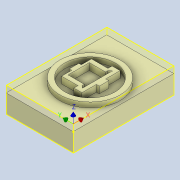
# Autodesk Inventor part: CNC#2 FInal
Saved by Autodesk Inventor 2022 (Build 260153000, 153)
## iProperties
Created: 2022-01-13
Part Number: CNC#2 FInal
Material: Generic
Document SubType Name: Modeling
Designer: student
Density: 1 g/cm^3
Appearance: Default
Author: student
Autodesk Inventor part; units mm, degrees
ref_plane "YZ Plane" through (0, 0, 0) normal (1, 0, 0) x (0, 1, 0)
ref_plane "XZ Plane" through (0, 0, 0) normal (0, 1, 0) x (-1, 0, 0)
ref_plane "XY Plane" through (0, 0, 0) normal (0, 0, 1) x (1, 0, 0)
sketch "Sketch1" plane through (0, 0, 0) normal (0, 1, 0) x (-1, 0, 0)
  line L0 (0, 0) -> (50.8, 0)
  line L1 (50.8, 0) -> (50.8, -76.2)
  line L2 (50.8, -76.2) -> (0, -76.2)
  line L3 (0, -76.2) -> (0, 0)
  dimension "d0" = 50.8
  dimension "d1" = 76.2
  constraints: 8 end point, 2 parallel, 1 horizontal, 1 perpendicular
  measures "d0" distance of L1.end L2.end
  measures "d1" distance of L0.end L1.end
extrude "Extrusion1" add sketch "Sketch1" along normal blind 13.97
sketch "Sketch6" plane through (0, 13.97, 0) normal (0, 1, 0) x (1, 0, 0)
  point P0 (0, 0)
sketch "Sketch7" plane through (0, 13.97, 0) normal (0, 1, 0) x (1, 0, 0)
  point P0 (0, 0)
sketch "Sketch8" plane through (0, 13.97, 0) normal (0, 1, 0) x (1, 0, 0)
  circle A0 centre (-25.4, 38.1) radius 22.86
  circle A1 centre (-25.4, 38.1) radius 19.05
  point P0 (0, 0)
  dimension "d30" = 45.72
  dimension "d31" = 38.1
  constraints: 2 centre point, 1 coincident
  measures "d30" diameter of A0
  measures "d31" diameter of A1
extrude "Extrusion15" add sketch "Sketch8" along normal blind 3.81
sketch "Sketch9" plane through (-25.4, 13.97, -38.1) normal (0, 1, 0) x (1, 0, 0)
  line L0 (-8.6694, 8.1535) -> (3.6792, 8.1535)
  line L1 (3.6792, 8.1535) -> (3.6792, 9.8977)
  line L2 (3.6792, 9.8977) -> (5.4931, 11.4325)
  line L3 (5.4931, 11.4325) -> (5.4931, 0.0971)
  line L4 (-8.6694, 8.1535) -> (-8.6694, 0.0971)
  line L5 (-8.6694, -7.9593) -> (3.6792, -7.9593)
  line L6 (3.6792, -7.9593) -> (3.6792, -9.7035)
  line L7 (3.6792, -9.7035) -> (5.4931, -11.2383)
  line L8 (5.4931, -11.2383) -> (5.4931, 0.0971)
  line L9 (-8.6694, -7.9593) -> (-8.6694, 0.0971)
  line L10 (8.2546, 0.0971) -> (8.2546, -14.3778)
  line L11 (8.2546, -14.3778) -> (2.1623, -14.3778)
  line L12 (2.1623, -14.3778) -> (2.1623, -11.2383)
  line L13 (2.1623, -11.2383) -> (-10.3102, -11.2383)
  line L14 (-10.3102, -11.2383) -> (-10.3102, 0.0971)
  line L15 (8.2546, 0.0971) -> (8.2546, 14.572)
  line L16 (8.2546, 14.572) -> (2.1623, 14.572)
  line L17 (2.1623, 14.572) -> (2.1623, 11.4325)
  line L18 (2.1623, 11.4325) -> (-10.3102, 11.4325)
  line L19 (-10.3102, 11.4325) -> (-10.3102, 0.0971)
  line L20 (-12.1685, 0.0971) -> (-12.1685, -3.512)
  line L21 (-12.1685, -3.512) -> (-10.3102, -3.512)
  line L22 (-10.3102, -3.512) -> (-10.3102, 0.0971)
  line L23 (-12.1685, 0.0971) -> (-12.1685, 3.7061)
  line L24 (-12.1685, 3.7061) -> (-10.3102, 3.7061)
  line L25 (10.4745, 0.0971) -> (10.4745, -3.512)
  line L26 (10.4745, -3.512) -> (8.2546, -3.512)
  line L27 (8.2546, -3.512) -> (8.2546, 0.0971)
  line L28 (10.4745, 0.0971) -> (10.4745, 3.7061)
  line L29 (10.4745, 3.7061) -> (8.2546, 3.7061)
  point P0 (25.4, -38.1)
  point P1 (8.2546, -3.512)
  point P2 (8.2546, 3.7061)
  point P3 (-10.3102, 3.7061)
  point P4 (-10.3102, -3.512)
  constraints: 60 end point, 5 perpendicular, 2 parallel, 2 vertical
extrude "Extrusion16" add sketch "Sketch9" along normal blind 5.08
body "Solid1"
